Autodesk Fusion 360 part; units mm, degrees
(part 11 of 11)
  arc A117 (-48.8956, 11.0425) -> (-49.1597, 9.7998) centre (0, 0) ccw
  spline S234 degree 5 poles (-49.1597, 9.7998) (-49.1483, 9.7916) (-49.1256, 9.7752) (-49.0914, 9.7506) (-49.0457, 9.718) (-48.9886, 9.6774) (-48.9314, 9.6371) (-48.874, 9.597) (-48.8166, 9.5571) (-48.7591, 9.5175) (-48.7015, 9.4781) (-48.6438, 9.4389) (-48.586, 9.4) (-48.5281, 9.3613) (-48.4702, 9.3229) (-48.4121, 9.2847) (-48.354, 9.2468) (-48.2957, 9.2091) (-48.2374, 9.1717) (-48.179, 9.1345) (-48.1205, 9.0975) (-48.0619, 9.0609) (-48.0032, 9.0245) (-47.9444, 8.9883) (-47.8855, 8.9524) (-47.8265, 8.9168) (-47.7674, 8.8815) (-47.7083, 8.8464) (-47.649, 8.8116) (-47.5897, 8.7771) (-47.5303, 8.7429) (-47.4707, 8.7089) (-47.4111, 8.6752) (-47.3514, 8.6419) (-47.2916, 8.6088) (-47.2317, 8.576) (-47.1717, 8.5435) (-47.1116, 8.5113) (-47.0514, 8.4795) (-46.9911, 8.4479) (-46.9307, 8.4167) (-46.8702, 8.3857) (-46.8096, 8.3552) (-46.7489, 8.3249) (-46.6882, 8.295) (-46.6273, 8.2654) (-46.5663, 8.2361) (-46.5052, 8.2073) (-46.4441, 8.1788) (-46.3828, 8.1506) (-46.3214, 8.1228) (-46.2599, 8.0954) (-46.2094, 8.0733) (-46.1711, 8.0567) (-46.1452, 8.0456) (-46.1316, 8.0398) (-46.1303, 8.0392) knots -1 -1 -1 -1 -1 -1 -0.985714 -0.971429 -0.957143 -0.942857 -0.928571 -0.914286 -0.9 -0.885714 -0.871429 -0.857143 -0.842857 -0.828571 -0.814286 -0.8 -0.785714 -0.771429 -0.757143 -0.742857 -0.728571 -0.714286 -0.7 -0.685714 -0.671429 -0.657143 -0.642857 -0.628571 -0.614286 -0.6 -0.585714 -0.571429 -0.557143 -0.542857 -0.528571 -0.514286 -0.5 -0.485714 -0.471429 -0.457143 -0.442857 -0.428571 -0.414286 -0.4 -0.385714 -0.371429 -0.357143 -0.342857 -0.328571 -0.314286 -0.3 -0.285714 -0.271429 -0.269981 -0.269981 -0.269981 -0.269981 -0.269981 -0.269981
  spline S235 degree 3 poles (-45.8928, 7.606) (-45.8843, 7.6574) (-45.8859, 7.7099) (-45.9091, 7.8115) (-45.9306, 7.8595) (-45.9819, 7.9322) (-46.0072, 7.9592) (-46.0646, 8.0056) (-46.0964, 8.0248) (-46.1303, 8.0392) knots 0 0 0 0 0.015626 0.015626 0.031252 0.031252 0.042323 0.042323 0.053393 0.053393 0.053393 0.053393
  arc A118 (-45.8928, 7.606) -> (-45.997, 6.9479) centre (0, 0) ccw
  spline S236 degree 3 poles (-46.3568, 6.6093) (-46.3049, 6.6139) (-46.2545, 6.6287) (-46.162, 6.6767) (-46.1209, 6.7095) (-46.0634, 6.7774) (-46.0436, 6.8087) (-46.0131, 6.8759) (-46.0025, 6.9115) (-45.997, 6.9479) knots 0 0 0 0 0.015626 0.015626 0.031252 0.031252 0.042323 0.042323 0.053393 0.053393 0.053393 0.053393
  spline S237 degree 5 poles (-46.3568, 6.6093) (-46.3582, 6.6092) (-46.3729, 6.6078) (-46.401, 6.6053) (-46.4425, 6.6013) (-46.4974, 6.5959) (-46.5644, 6.5888) (-46.6313, 6.5814) (-46.6983, 6.5735) (-46.7653, 6.5653) (-46.8323, 6.5567) (-46.8993, 6.5478) (-46.9664, 6.5385) (-47.0334, 6.5288) (-47.1005, 6.5187) (-47.1676, 6.5084) (-47.2346, 6.4977) (-47.3017, 6.4866) (-47.3688, 6.4752) (-47.4359, 6.4635) (-47.503, 6.4515) (-47.5701, 6.4391) (-47.6372, 6.4265) (-47.7043, 6.4135) (-47.7714, 6.4002) (-47.8385, 6.3866) (-47.9056, 6.3727) (-47.9728, 6.3585) (-48.0399, 6.344) (-48.107, 6.3292) (-48.1741, 6.3142) (-48.2412, 6.2988) (-48.3083, 6.2832) (-48.3754, 6.2672) (-48.4424, 6.251) (-48.5095, 6.2345) (-48.5766, 6.2178) (-48.6436, 6.2007) (-48.7107, 6.1834) (-48.7777, 6.1658) (-48.8448, 6.148) (-48.9118, 6.1299) (-48.9788, 6.1115) (-49.0458, 6.0929) (-49.1128, 6.074) (-49.1798, 6.0548) (-49.2468, 6.0354) (-49.3137, 6.0157) (-49.3807, 5.9958) (-49.4476, 5.9756) (-49.5145, 5.9552) (-49.5814, 5.9345) (-49.6483, 5.9136) (-49.7018, 5.8967) (-49.7419, 5.8839) (-49.7686, 5.8753) (-49.782, 5.871) knots 0.269981 0.269981 0.269981 0.269981 0.269981 0.269981 0.271429 0.285714 0.3 0.314286 0.328571 0.342857 0.357143 0.371429 0.385714 0.4 0.414286 0.428571 0.442857 0.457143 0.471429 0.485714 0.5 0.514286 0.528571 0.542857 0.557143 0.571429 0.585714 0.6 0.614286 0.628571 0.642857 0.657143 0.671429 0.685714 0.7 0.714286 0.728571 0.742857 0.757143 0.771429 0.785714 0.8 0.814286 0.828571 0.842857 0.857143 0.871429 0.885714 0.9 0.914286 0.928571 0.942857 0.957143 0.971429 0.985714 1 1 1 1 1 1
  arc A119 (-49.782, 5.871) -> (-49.9148, 4.6076) centre (0, 0) ccw
  spline S238 degree 5 poles (-49.9148, 4.6076) (-49.9026, 4.6006) (-49.8782, 4.5866) (-49.8417, 4.5657) (-49.7929, 4.5381) (-49.7318, 4.5037) (-49.6707, 4.4696) (-49.6094, 4.4357) (-49.5482, 4.402) (-49.4868, 4.3686) (-49.4254, 4.3355) (-49.364, 4.3026) (-49.3024, 4.2699) (-49.2408, 4.2375) (-49.1792, 4.2053) (-49.1174, 4.1734) (-49.0556, 4.1418) (-48.9938, 4.1104) (-48.9319, 4.0792) (-48.8699, 4.0484) (-48.8078, 4.0178) (-48.7457, 3.9874) (-48.6835, 3.9573) (-48.6213, 3.9275) (-48.559, 3.898) (-48.4966, 3.8687) (-48.4341, 3.8398) (-48.3716, 3.8111) (-48.3091, 3.7827) (-48.2464, 3.7545) (-48.1838, 3.7267) (-48.121, 3.6992) (-48.0582, 3.6719) (-47.9953, 3.645) (-47.9324, 3.6183) (-47.8694, 3.592) (-47.8063, 3.5659) (-47.7432, 3.5402) (-47.68, 3.5148) (-47.6167, 3.4897) (-47.5534, 3.465) (-47.49, 3.4405) (-47.4265, 3.4164) (-47.363, 3.3927) (-47.2995, 3.3693) (-47.2358, 3.3462) (-47.1721, 3.3235) (-47.1084, 3.3012) (-47.0446, 3.2792) (-46.9807, 3.2576) (-46.9167, 3.2364) (-46.8527, 3.2156) (-46.8001, 3.1989) (-46.7604, 3.1864) (-46.7334, 3.178) (-46.7193, 3.1737) (-46.718, 3.1733) knots -1 -1 -1 -1 -1 -1 -0.985714 -0.971429 -0.957143 -0.942857 -0.928571 -0.914286 -0.9 -0.885714 -0.871429 -0.857143 -0.842857 -0.828571 -0.814286 -0.8 -0.785714 -0.771429 -0.757143 -0.742857 -0.728571 -0.714286 -0.7 -0.685714 -0.671429 -0.657143 -0.642857 -0.628571 -0.614286 -0.6 -0.585714 -0.571429 -0.557143 -0.542857 -0.528571 -0.514286 -0.5 -0.485714 -0.471429 -0.457143 -0.442857 -0.428571 -0.414286 -0.4 -0.385714 -0.371429 -0.357143 -0.342857 -0.328571 -0.314286 -0.3 -0.285714 -0.271429 -0.269981 -0.269981 -0.269981 -0.269981 -0.269981 -0.269981
  spline S239 degree 3 poles (-46.4364, 2.7672) (-46.4333, 2.8192) (-46.4404, 2.8713) (-46.4742, 2.9699) (-46.5005, 3.0154) (-46.5591, 3.0823) (-46.5872, 3.1066) (-46.6491, 3.1467) (-46.6827, 3.1624) (-46.718, 3.1733) knots 0 0 0 0 0.015626 0.015626 0.031252 0.031252 0.042323 0.042323 0.053393 0.053393 0.053393 0.053393
  circle A120 centre (0, 0) radius 17.65
  circle A121 centre (0, 0) radius 38
  dimension "d12" = 76
  constraint concentric A0 A121
  measures "d12" diameter of A121
extrude "Extrude4" cut sketch "Sketch2 (2)" against normal blind 10 contours A121 in component "Spur Gear (60 teeth)"
sketch "Sketch3 (2)" plane through (0, 0, 5) normal (0, 0, 1) x (-1, 0, 0)
  circle A0 centre (0, 0) radius 17.65
  circle A1 centre (0, 0) radius 38
  circle A2 centre (0, 0) radius 22.5
  dimension "d16" = 45
  constraint coincident A0.centre A1.centre
  measures "d16" diameter of A2
extrude "Extrude5" add sketch "Sketch3 (2)" along normal blind 6 contours A2 in component "Spur Gear (60 teeth)"
component "Spur Gear (60 teeth)" placed x (1, 0, 0) y (0, 1, 0) z (0, 0, 1) at (0, 0, 0)
